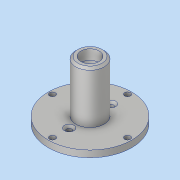
# Autodesk Inventor part: MotorMount
Saved by Autodesk Inventor 2017 (Build 210142000, 142)
## iProperties
Created: 2016-10-13
Part Number: MotorMount
Material: Generic
Document SubType Name: Modeling
Designer: techn
Density: 1 g/cm^3
Appearance: Aluminum - Flat
Author: techn
Autodesk Inventor part; units mm, degrees
ref_plane "YZ Plane" through (0, 0, 0) normal (1, 0, 0) x (0, 1, 0)
ref_plane "XZ Plane" through (0, 0, 0) normal (0, 1, 0) x (-1, 0, 0)
ref_plane "XY Plane" through (0, 0, 0) normal (0, 0, 1) x (1, 0, 0)
sketch "Sketch1" plane through (0, 0, 0) normal (0, 0, 1) x (1, 0, 0)
  line L0 (0, 0) -> (25, 0)
  line L1 (25, 0) -> (25, 4)
  line L2 (25, 4) -> (8.5, 4)
  line L3 (8.5, 4) -> (8.5, 35)
  line L4 (8.5, 35) -> (0, 35)
  line L5 (0, 0) -> (6.5, 0)
  line L6 (6.5, 0) -> (6.5, 29)
  line L7 (6.5, 29) -> (5.5, 29)
  line L8 (5.5, 29) -> (5.5, 35)
  line L9 (0, 35) -> (0, 0)
  dimension "d0" = 25
  dimension "d1" = 4
  dimension "d2" = 8.5
  dimension "d3" = 31
  dimension "d4" = 6.5
  dimension "d5" = 29
  dimension "d6" = 5.5
  constraints: 20 end point, 5 perpendicular, 3 horizontal, 2 point on line, 1 parallel
  measures "d0" distance of L0.start L0.end
  measures "d1" distance of L0.end L1.end
  measures "d2" horizontal distance of L0.start L2.end
  measures "d3" distance of L2.end L3.end
  measures "d4" distance of L0.start L5.end
  measures "d5" distance of L5.end L6.end
  measures "d6" horizontal distance of L7.end L0.start
revolve "Revolution1" add sketch "Sketch1" angle 360 about axis through (0, 35, 0) along (0, -1, 0) contours L6 L7 L8 L4 L3 L2 L1 L0
sketch "Sketch2" plane through (0, 4, 0) normal (0, 1, 0) x (1, 0, 0)
  circle A0 centre (0, -22.5) radius 1.75
  circle A1 centre (22.5, 0) radius 1.75
  circle A2 centre (0, 22.5) radius 1.75
  circle A3 centre (-22.5, 0) radius 1.75
  circle A4 centre (0, -12.5) radius 1.6
  circle A5 centre (0, 12.5) radius 1.6
  point P0 (0, 0)
  dimension "d8" = 3.5
  dimension "d9" = 22.5
  dimension "d12" = 360
  dimension "d14" = 3.2
  dimension "d15" = 12.5
  dimension "d18" = 360
  constraints: 6 centre point, 14 other
  measures "d8" diameter of A0
  measures "d9" distance of A0.centre point (0, 0)
  measures "d14" diameter of A4
  measures "d15" distance of point (0, 0) A4.centre
extrude "Extrusion1" cut sketch "Sketch2" against normal blind 25.4
chamfer "Chamfer1" distance 1.27 angle 45 2 edges at (-1.6, 4, 12.5) (-1.6, 4, -12.5)
chamfer "Chamfer2" distance 1.27 angle 45 1 edges at (-8.5, 35, 0)
body "Solid1"
